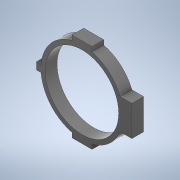
# Autodesk Inventor part: celestronTubeBracket
Saved by Autodesk Inventor 2021.2 (Build 252289000, 289)
## iProperties
Created: 2020-07-21
Part Number: celestronTubeBracket
Material: Aluminum 6061
Document SubType Name: Modeling
Designer: robst
Density: 2.7 g/cm^3
Appearance: Smooth - Black
Mass: 501.045 g
Surface Area: 442.424 cm^2
Volume: 185.572 cm^3
Author: robst
Autodesk Inventor part; units mm, degrees
ref_plane "YZ Plane" through (0, 0, 0) normal (1, 0, 0) x (0, 1, 0)
ref_plane "XZ Plane" through (0, 0, 0) normal (0, 1, 0) x (-1, 0, 0)
ref_plane "XY Plane" through (0, 0, 0) normal (0, 0, 1) x (1, 0, 0)
sketch "Sketch1" plane through (0, 0, 0) normal (0, 0, 1) x (1, 0, 0)
  circle A0 centre (0, 0) radius 79.375
  line L0 (82.5402, 33.02) -> (107.9402, 33.02)
  line L1 (107.9402, 33.02) -> (107.9402, 0)
  line L2 (-88.5728, 7.62) -> (-98.7328, 7.62)
  line L3 (-98.7328, 7.62) -> (-98.7328, 0)
  line L4 (0, 96.3985) -> (21.59, 96.3985)
  line L5 (21.59, 96.3985) -> (21.59, 86.2385)
  line L6 (82.5402, -33.02) -> (107.9402, -33.02)
  line L7 (107.9402, -33.02) -> (107.9402, 0)
  line L8 (-88.5728, -7.62) -> (-98.7328, -7.62)
  line L9 (-98.7328, -7.62) -> (-98.7328, 0)
  line L10 (0, 96.3985) -> (-21.59, 96.3985)
  line L11 (-21.59, 96.3985) -> (-21.59, 86.2385)
  arc A1 (-88.5728, -7.62) -> (-21.59, -86.2385) centre (0, 0) ccw
  arc A2 (-21.59, 86.2385) -> (-88.5728, 7.62) centre (0, 0) ccw
  arc A3 (21.59, -86.2385) -> (82.5402, -33.02) centre (0, 0) ccw
  arc A4 (82.5402, 33.02) -> (21.59, 86.2385) centre (0, 0) ccw
  line L12 (-88.9, 0) -> (88.9, 0) construction
  line L13 (0, -96.3985) -> (21.59, -96.3985)
  line L14 (21.59, -96.3985) -> (21.59, -86.2385)
  line L15 (0, -96.3985) -> (-21.59, -96.3985)
  line L16 (-21.59, -96.3985) -> (-21.59, -86.2385)
  arc A5 (-21.59, 86.2385) -> (-88.5728, 7.62) centre (0, 0) ccw
  arc A6 (82.5402, 33.02) -> (21.59, 86.2385) centre (0, 0) ccw
  arc A7 (-88.5728, -7.62) -> (-21.59, -86.2385) centre (0, 0) ccw
  arc A8 (21.59, -86.2385) -> (82.5402, -33.02) centre (0, 0) ccw
  dimension "d2" = 25.4
  dimension "d5" = 10.16
  dimension "d7" = 10.16
  dimension "d8" = 7.62
  dimension "d10" = 33.02
  dimension "d13" = 21.59
  dimension "d14" = 158.75
  dimension "d15" = 177.8
  constraints: 34 end point, 16 point on circle, 9 centre point, 4 horizontal, 3 coincident, 3 perpendicular, 3 symmetric about line
  measures "d2" distance of L0.start L0.end
  measures "d5" distance of L4.end L5.end
  measures "d7" distance of L2.start L2.end
  measures "d8" distance of L2.end L3.end
  measures "d10" distance of L0.end L1.end
  measures "d13" distance of L4.start L4.end
  measures "d14" diameter of A0
  measures "d15" diameter of A2
extrude "Extrusion2" add sketch "Sketch1" along normal mid plane 25.4
body "Solid2"
